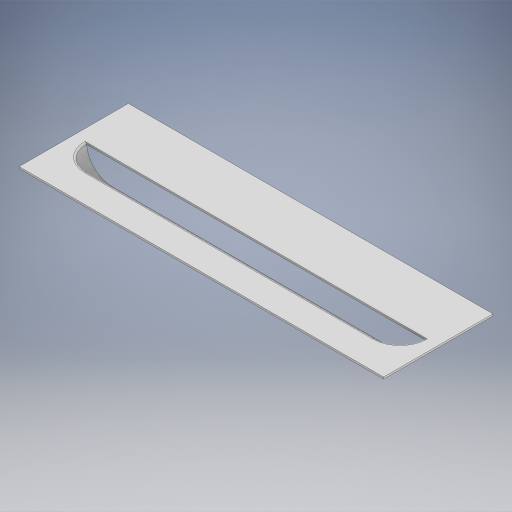
# Autodesk Inventor part: A2.3-punch
Saved by Autodesk Inventor 2024 (Build 280153000, 153)
## iProperties
Created: 2024-02-08
Part Number: A2.3-punch
Material: Generic
Document SubType Name: Sheet Metal
Designer: Alex
Density: 1 g/cm^3
Sheet Metal Rule: Default_mm
Appearance: Default
Author: Alex
Autodesk Inventor part; units mm, degrees
ref_plane "YZ Plane" through (0, 0, 0) normal (1, 0, 0) x (0, 1, 0)
ref_plane "XZ Plane" through (0, 0, 0) normal (0, 1, 0) x (-1, 0, 0)
sketch "Sketch1" plane through (0, 0, 0) normal (0, 1, 0) x (-1, 0, 0)
  line L0 (0, 0) -> (-100, 0)
  line L1 (-100, 0) -> (-100, -30)
  line L2 (-100, -30) -> (0, -30)
  line L3 (0, -30) -> (0, 0)
  dimension "d0" = 100
  dimension "d1" = 30
  measures "d0" distance of L1.end L2.end
  measures "d1" distance of L0.end L1.end
extrude "Plate1" add sketch "Sketch1" along normal blind 0.5
sketch "Sketch2" plane through (0, 0.5, 0) normal (0, 1, 0) x (1, 0, 0)
  arc A0 (3.5, 15) -> (10.5, 8) centre (10.5, 15) ccw
  line L0 (10.5, 8) -> (89.5, 8)
  arc A1 (89.5, 8) -> (96.5, 15) centre (89.5, 15) ccw
  line L1 (3.5, 15) -> (96.5, 15)
  line L2 (50, 15) -> (50, 8) construction
  line L3 (100, 0) -> (0, 0) construction
  line L4 (0, 0) -> (0, 30) construction
  dimension "d3" = 93
  dimension "d4" = 7
  dimension "d5" = 15
  dimension "d6" = 50
  constraints: 6 end point, 4 point on circle, 2 centre point, 2 horizontal, 2 midpoint, 2 point on line, 1 coincident, 1 equal radius, 1 tangent
  measures "d3" distance of L1.start L1.end
  measures "d4" radius of A0
  measures "d5" distance from line of L3 point (50, 15)
  measures "d6" distance from line of L4 point (50, 15)
extrude "Extrusion1" cut sketch "Sketch2" against normal blind 0.5
ref_plane "Work Plane1" through (26.75, 0.5, -15) normal (0, -1, 0) x (1, 0, 0)
sketch "Sketch3" plane through (26.75, 0.5, -15) normal (0, -1, 0) x (1, 0, 0)
  arc A0 (-16.25, 7) -> (-23.25, 0) centre (-16.25, 0) ccw projected
  line L0 (-23.25, 0) -> (69.75, 0) projected
  line L1 (62.75, 7) -> (-16.25, 7) projected
  arc A1 (69.75, 0) -> (62.75, 7) centre (62.75, 0) ccw projected
  line L2 (23.25, 0) -> (23.25, 7) construction
  line L3 (69.75, 0) -> (-23.25, 0) projected
  line L4 (-23.25, 0) -> (-23.75, 0)
  arc A2 (-16.25, 7.5) -> (-23.75, 0) centre (-16.25, 0) ccw
  line L5 (-16.25, 7.5) -> (62.75, 7.5)
  arc A3 (70.25, 0) -> (62.75, 7.5) centre (62.75, 0) ccw
  line L6 (70.25, 0) -> (69.75, 0)
  point P0 (-26.75, 15)
  dimension "d9" = 0.5
  constraints: 6 end point, 4 point on circle, 2 centre point, 2 concentric, 2 horizontal, 2 tangent, 1 point on line
  measures "d9" distance of L0.start L4.end
revolve "Revolution1" add sketch "Sketch3" angle 90 about axis through (3.5, 0.5, -15) along (1, 0, 0) contours A0 L4 A2 L5 A3 L6 A1 L1
fillet "Fillet2" radius 0.5 6 edges at (94.7915, 0, -9.7085) (5.2085, 0, -9.7085) (50, 0, -7.5167) (5.5503, 0.5, -10.0503) (94.4497, 0.5, -10.0503) (50, 0.5, -8)
equation "\"d7\" = Thickness"
equation "\"d9\" = Thickness"
equation "\"d2\" = Thickness"
equation "\"BendRadius\" = Thickness"
equation "\"BendReliefWidth\" = Thickness"
equation "\"BendReliefDepth\" = 0.5 * Thickness"
equation "\"CornerReliefSize\" = 4 * Thickness"
equation "\"MinimumRemnant\" = 2 * Thickness"
equation "\"TransitionRadius\" = BendRadius"
equation "\"JacobiRadiusSize\" = BendRadius"
equation "\"GapSize\" = Thickness"
equation "\"Thickness\" = 0.5"
body "Solid1"
